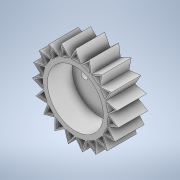
# Autodesk Inventor part: Antriebsrad
Saved by Autodesk Inventor 2021 (Build 250183000, 183)
## iProperties
Created: 2024-05-10
Part Number: Antriebsrad
Material: Generic
Document SubType Name: Modeling
Designer: Lukas
Density: 1 g/cm^3
Appearance: Default
Author: Lukas
Autodesk Inventor part; units mm, degrees
ref_plane "YZ Plane" through (0, 0, 0) normal (1, 0, 0) x (0, 1, 0)
ref_plane "XZ Plane" through (0, 0, 0) normal (0, 1, 0) x (-1, 0, 0)
ref_plane "XY Plane" through (0, 0, 0) normal (0, 0, 1) x (1, 0, 0)
sketch "Sketch1" plane through (0, 0, 0) normal (0, 0, 1) x (1, 0, 0)
  circle A0 centre (0, 0) radius 9.05
  circle A1 centre (0, 0) radius 10.55
  line L0 (-2, 10.15) -> (0, 14)
  line L1 (0, 14) -> (2, 10.15)
  line L2 (2, 10.15) -> (-2, 10.15)
  line L3 (-1.3415, 10.55) -> (0, 13.1323)
  line L4 (0, 13.1323) -> (1.3415, 10.55)
  line L5 (1.3415, 10.55) -> (-1.3415, 10.55)
  circle A2 centre (-5, 0) radius 1.1
  circle A3 centre (5, 0) radius 1.1
  circle A4 centre (0, 0) radius 1.25
  point P0 (0, 10.55)
  point P1 (0, 10.15)
  point P2 (0, 10.55)
  point P3 (1.8799, 10.3812)
  point P4 (-1.8799, 10.3812)
  dimension "d0" = 18.1
  dimension "d1" = 1.5
  dimension "d17" = 10.55
  dimension "d18" = 14
  dimension "d19" = 0.4
  dimension "d20" = 0.4
  dimension "d21" = 4
  dimension "d22" = 10
  dimension "d23" = 5
  dimension "d24" = 2.2
  dimension "d25" = 2.5
  constraints: 12 end point, 5 centre point, 4 vertical alignment, 3 coincident, 3 parallel, 2 horizontal alignment, 2 midpoint, 1 equal radius, 1 horizontal
  measures "d0" diameter of A0
  measures "d1" radial gap between concentric circles of A1 A0
  measures "d17" distance from line of point (0, 0) L5
  measures "d18" distance of point (0, 0) L0.end
  measures "d19" distance between parallel lines of L0 L3
  measures "d20" distance between parallel lines of L2 L5
  measures "d21" distance of L1.end L0.start
  measures "d22" distance of A3.centre A2.centre
  measures "d23" distance of point (0, 0) A2.centre
  measures "d24" diameter of A2
  measures "d25" diameter of A4
extrude "Extrusion1" add sketch "Sketch1" along normal blind 1.5 contours A0 | A1 L0 L2 L1 | L1 L2 L0 A1
extrude "Extrusion2" add sketch "Sketch1" along normal blind 9.5 contours A1 L0 L2 L1 | L1 L2 L0 A1
extrude "Extrusion3" add sketch "Sketch1" along normal up to surface (9.5 mm away) contours A1 L0 L1
pattern_circular "Circular Pattern1" count 19 over 360 about axis through (0, 0, 0) along (0, 0, 1) of "Extrusion3"
equation "\"d17\" = 0.5 * d0 + d1"
equation "\"d20\" = d19"
equation "\"d23\" = 0.5 * d22"
body "Solid1"
